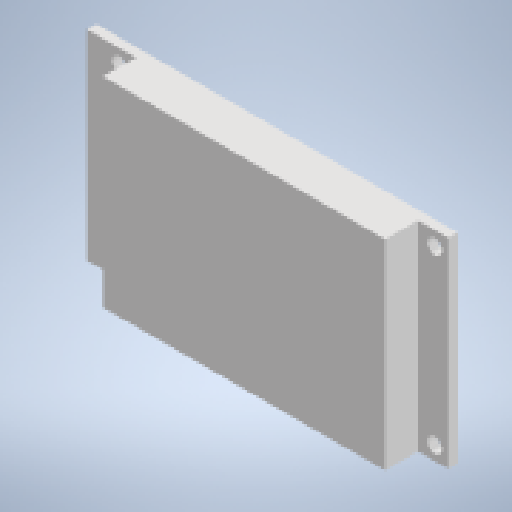
# Autodesk Inventor part: Ecran
Saved by Autodesk Inventor 2023 (Build 270158000, 158)
## iProperties
Created: 2023-04-14
Part Number: Ecran
Material: Glass
Document SubType Name: Modeling
Designer: Timothée
Density: 2.18 g/cm^3
Appearance: Clear
Author: Timothée
Autodesk Inventor part; units mm, degrees
ref_plane "YZ Plane" through (0, 0, 0) normal (1, 0, 0) x (0, 1, 0)
ref_plane "XZ Plane" through (0, 0, 0) normal (0, 1, 0) x (-1, 0, 0)
ref_plane "XY Plane" through (0, 0, 0) normal (0, 0, 1) x (1, 0, 0)
sketch "Ecran" plane through (0, 0, 0) normal (0, 0, 1) x (1, 0, 0)
  line L0 (-38.59, 21.36) -> (38.59, 21.36)
  line L1 (38.59, 21.36) -> (38.59, 0)
  line L2 (-38.59, 0) -> (-38.59, 21.36)
  circle A0 centre (35.59, 18.36) radius 1.6
  line L3 (-38.59, 0) -> (38.59, 0)
  line L4 (35.59, 21.36) -> (35.59, 0)
  line L5 (-31.67, 21.36) -> (-31.67, 0)
  circle A1 centre (-31.67, 18.36) radius 1.6
  line L6 (-38.59, -21.36) -> (38.59, -21.36)
  line L7 (38.59, -21.36) -> (38.59, 0)
  line L8 (-38.59, 0) -> (-38.59, -21.36)
  circle A2 centre (35.59, -18.36) radius 1.6
  line L9 (35.59, -21.36) -> (35.59, 0)
  line L10 (-31.67, -21.36) -> (-31.67, 0)
  circle A3 centre (-31.67, -18.36) radius 1.6
  line L11 (32.08, 21.36) -> (-28.18, 21.36)
  line L12 (-28.18, 21.36) -> (-28.18, -21.36)
  line L13 (-28.18, -21.36) -> (32.08, -21.36)
  line L14 (32.08, -21.36) -> (32.08, 21.36)
  point P0 (0, 0)
  point P1 (38.59, 10.68)
  point P2 (35.59, 10.68)
  point P3 (38.59, -10.68)
  point P4 (35.59, -10.68)
  dimension "d3" = 3.2
  dimension "d4" = 3
  dimension "d5" = 77.18
  dimension "d6" = 21.36
  dimension "d8" = 67.26
  dimension "d9" = 3
  dimension "d12" = 60.26
  dimension "d13" = 6.51
  constraints: 30 end point, 12 point on line, 8 symmetric about line, 4 centre point, 3 parallel, 3 perpendicular, 2 horizontal, 2 midpoint, 2 other
  measures "d3" diameter of A0
  measures "d4" distance from line of L0 A0.centre
  measures "d5" distance of L0.start L0.end
  measures "d6" distance of L0.end L1.end
  measures "d8" distance between parallel lines of L4 L5
  measures "d9" distance of point (38.59, 10.68) point (35.59, 10.68)
  measures "d12" distance of L13.end L12.end
  measures "d13" distance between parallel lines of L7 L14
extrude "Extrusion1" add sketch "Ecran" along normal blind 9 contours L0 L5 A1 L3 L2 | L0 L12 L3 L5 A1 | L3 L10 A3 L6 L8 | L0 L14 L3 L12 | L3 L12 L6 L10 A3 | L0 L4 A0 L3 L14 | L3 L14 L6 L12 | L0 L1 L3 L4 A0 | L3 L9 A2 L6 L14 | L3 L7 L6 L9 A2
sketch "Sketch3" plane through (0, 0, 9) normal (0, 0, 1) x (1, 0, 0)
  line L0 (38.59, 21.36) -> (-38.59, 21.36) projected
  line L1 (-38.59, -21.36) -> (38.59, -21.36) projected
  line L2 (38.59, 21.36) -> (32.08, 21.36)
  line L3 (32.08, 21.36) -> (32.08, -21.36)
  line L4 (32.08, -21.36) -> (38.59, -21.36)
  line L5 (38.59, -21.36) -> (38.59, 21.36)
  line L6 (32.08, -21.36) -> (-28.18, -21.36)
  line L7 (-28.18, -21.36) -> (-28.18, 21.36)
  line L8 (-28.18, 21.36) -> (32.08, 21.36)
  line L9 (32.08, 21.36) -> (32.08, -21.36)
  line L10 (-38.59, 21.36) -> (-38.59, -21.36) projected
  line L11 (-28.18, 21.36) -> (-38.59, 21.36)
  line L12 (-38.59, 21.36) -> (-38.59, -21.36)
  line L13 (-38.59, -21.36) -> (-28.18, -21.36)
  line L14 (-28.18, -21.36) -> (-28.18, 21.36)
  point P0 (0, 0)
  point P1 (38.59, -21.36)
  dimension "d14" = 6.51
  dimension "d15" = 60.26
  constraints: 24 end point, 6 parallel, 3 horizontal, 3 perpendicular, 2 point on line
  measures "d14" distance of L4.end L3.end
  measures "d15" distance of L7.end L8.end
extrude "Extrusion2" cut sketch "Sketch3" against normal blind 7 contours L5 L1 L3 L0 | L7 L1 L10 L0
body "Solid1"
